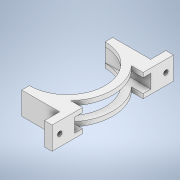
# Autodesk Inventor part: LensSupport
Saved by Autodesk Inventor 2022.2 (Build 262287010, 287A)
## iProperties
Created: 2022-05-11
Part Number: LensSupport
Material: Plástico ABS
Document SubType Name: Modeling
Designer: mabel
Density: 1.06 g/cm^3
Appearance: Suave - Blanco
Author: mabel
Autodesk Inventor part; units mm, degrees
ref_plane "YZ Plane" through (0, 0, 0) normal (1, 0, 0) x (0, 1, 0)
ref_plane "XZ Plane" through (0, 0, 0) normal (0, 1, 0) x (-1, 0, 0)
ref_plane "XY Plane" through (0, 0, 0) normal (0, 0, 1) x (1, 0, 0)
sketch "Boceto1" plane through (0, 0, 0) normal (0, 1, 0) x (-1, 0, 0)
  arc A0 (0, 25) -> (0, -25) centre (0, 0) ccw
  arc A1 (0, 30) -> (0, -30) centre (0, 0) ccw
  line L0 (0, 30) -> (-30, 30)
  line L1 (-30, 30) -> (-30, 20)
  line L2 (-30, 20) -> (-22.3607, 20)
  line L3 (0, 0) -> (-6.35, 0) construction
  line L4 (0, -30) -> (-30, -30)
  line L5 (-30, -30) -> (-30, -20)
  line L6 (-30, -20) -> (-22.3607, -20)
  line L7 (0, 30) -> (0, 25)
  line L8 (0, -25) -> (0, -30)
  dimension "d0" = 50
  dimension "d1" = 5
  dimension "d2" = 10
  constraints: 18 end point, 5 point on circle, 4 symmetric about line, 2 centre point, 2 horizontal, 2 perpendicular, 2 vertical, 1 coincident, 1 tangent
  measures "d0" diameter of A0
  measures "d1" radial gap between concentric circles of A0 A1
  measures "d2" distance of L0.end L1.end
extrude "Extrusión1" add sketch "Boceto1" along normal blind 15
sketch "Boceto2" plane through (0, 0, 25) normal (-1, 0, 0) x (0, 0, 1)
  line L0 (-25, 0) -> (-25, 27.7838) construction
  line L1 (0, 12.05) -> (-50, 12.05)
  line L2 (0, 2.95) -> (-50, 2.95)
  line L3 (-50, 2.95) -> (-50.15, 2.95)
  line L4 (-50.15, 2.95) -> (-50.15, 12.05)
  line L5 (-50.15, 12.05) -> (-50, 12.05)
  line L6 (0, 2.95) -> (0.15, 2.95)
  line L7 (0.15, 2.95) -> (0.15, 12.05)
  line L8 (0.15, 12.05) -> (0, 12.05)
  dimension "d19" = 0.15
  constraints: 18 end point, 4 symmetric about line, 1 horizontal, 1 vertical
  measures "d19" distance of L2.end L3.end
extrude "Extrusión2" cut sketch "Boceto2" against normal blind 25
sketch "Boceto3" plane through (25, 0, 25) normal (-1, 0, 0) x (0, 0, 1)
  line L0 (-50, 2.95) -> (-50.15, 2.95) projected
  line L1 (0.15, 12.05) -> (0.15, 2.95) projected
  line L2 (-50.15, 2.95) -> (-50.15, 12.05) projected
  line L3 (0.15, 12.05) -> (-50.15, 12.05)
  line L4 (-50.15, 12.05) -> (-50.15, 2.95)
  line L5 (-50.15, 2.95) -> (0.15, 2.95)
  line L6 (0.15, 2.95) -> (0.15, 12.05)
  point P0 (-25, 0)
  point P1 (-41.5831, 2.95)
  point P2 (2, 12.05)
  point P3 (-52, 2.95)
  point P4 (-51, 2.95)
  point P5 (1, 12.05)
  point P6 (0.15, 2.95)
  constraints: 8 end point, 2 parallel, 1 horizontal, 1 perpendicular
extrude "Extrusión3" cut sketch "Boceto3" against normal blind 25
sketch "Boceto4" plane through (30, 0, -30) normal (0, 0, -1) x (-1, 0, 0)
  line L0 (0, 0) -> (0, 2.95) projected
  line L1 (7.6393, 15) -> (0, 15) projected
  line L2 (0, 0) -> (5, 0)
  line L3 (5, 0) -> (5, 15)
  line L4 (5, 15) -> (0, 15)
  line L5 (0, 15) -> (0, 0)
  point P0 (30, 0)
  dimension "d12" = 5
  constraints: 8 end point, 2 parallel, 2 point on line, 1 horizontal, 1 perpendicular
  measures "d12" distance of L4.end L3.end
extrude "Extrusión4" add sketch "Boceto4" along normal blind 10
mirror "Simetría1" about plane through (0, 0, 0) normal (0, 0, 1) of "Extrusión4"
sketch "Boceto6" plane through (25, 0, -30) normal (-1, 0, 0) x (0, 0, 1)
  line L0 (0, 15) -> (-10, 15) projected
  line L1 (-10, 0) -> (-10, 15) projected
  line L2 (0, 15) -> (-10, 15)
  line L3 (-10, 15) -> (-10, 0)
  line L4 (-10, 0) -> (0, 0)
  line L5 (0, 0) -> (0, 15)
  circle A0 centre (-5, 7.5) radius 1.5
  point P0 (30, 0)
  dimension "d15" = 3
  constraints: 8 end point, 2 parallel, 1 centre point, 1 horizontal, 1 perpendicular
  measures "d15" diameter of A0
extrude "Extrusión5" cut sketch "Boceto6" against normal blind 10 contours A0
mirror "Simetría2" about plane through (0, 0, 0) normal (0, 0, 1) of "Extrusión5"
